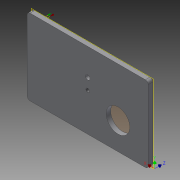
# Autodesk Inventor part: capac
Saved by Autodesk Inventor 2015 SP1 (Build 190203100, 203)
## iProperties
Created: 2015-04-26
Part Number: capac
Material: Generic
Document SubType Name: Modeling
Designer: ubik
Density: 1 g/cm^3
Appearance: Default
Author: ubik
Autodesk Inventor part; units mm, degrees
ref_plane "YZ Plane" through (0, 0, 0) normal (1, 0, 0) x (0, 1, 0)
ref_plane "XZ Plane" through (0, 0, 0) normal (0, 1, 0) x (-1, 0, 0)
ref_plane "XY Plane" through (0, 0, 0) normal (0, 0, 1) x (1, 0, 0)
ref_plane "Work Plane1" through (0, -1.5067, 123.4533) normal (0, 0, 1) x (1, 0, 0)
sketch "Sketch1" plane through (0, -1.5067, 123.4533) normal (0, 0, 1) x (1, 0, 0)
  arc A0 (-98.75, -51) -> (-86.75, -63) centre (-86.75, -51) ccw projected
  line L0 (86.75, -63) -> (-86.75, -63) projected
  arc A1 (86.75, -63) -> (98.75, -51) centre (86.75, -51) ccw projected
  line L1 (98.75, 51) -> (98.75, -51) projected
  arc A2 (98.75, 51) -> (86.75, 63) centre (86.75, 51) ccw projected
  line L2 (-86.75, 63) -> (86.75, 63) projected
  arc A3 (-86.75, 63) -> (-98.75, 51) centre (-86.75, 51) ccw projected
  line L3 (-98.75, -51) -> (-98.75, 51) projected
  line L4 (93.75, 46) -> (93.75, -46) projected
  arc A4 (81.75, -58) -> (93.75, -46) centre (81.75, -46) ccw projected
  line L5 (81.75, -58) -> (-81.75, -58) projected
  arc A5 (-93.75, -46) -> (-81.75, -58) centre (-81.75, -46) ccw projected
  line L6 (-93.75, -46) -> (-93.75, 46) projected
  arc A6 (-81.75, 58) -> (-93.75, 46) centre (-81.75, 46) ccw projected
  line L7 (-81.75, 58) -> (81.75, 58) projected
  arc A7 (93.75, 46) -> (81.75, 58) centre (81.75, 46) ccw projected
  point P0 (0, 1.5067)
sketch "Sketch2" plane through (0, -1.5067, 123.4533) normal (0, 0, 1) x (1, 0, 0)
  line L0 (-107.5, 69.0067) -> (107.5, 69.0067)
  line L1 (107.5, 69.0067) -> (107.5, -65.9933)
  line L2 (107.5, -65.9933) -> (-107.5, -65.9933)
  line L3 (-107.5, -65.9933) -> (-107.5, 69.0067)
  point P0 (0, 1.5067)
  dimension "height" = 135
  dimension "width" = 215
  dimension "d2" = 107.5
  dimension "d3" = 67.5
  constraints: 8 end point, 2 parallel, 1 horizontal, 1 perpendicular
  measures "height" distance of L2.end L0.start
  measures "width" distance of L0.start L0.end
  measures "d2" distance from line of point (0, 1.507) L3
  measures "d3" distance from line of point (0, 1.507) L2
extrude "Extrusion1" add sketch "Sketch2" along normal blind 8
fillet "Fillet1" radius 5 4 edges at (-107.5, 67.5, 127.4533) (107.5, 67.5, 127.4533) (107.5, -67.5, 127.4533) (-107.5, -67.5, 127.4533)
extrude "Extrusion2" cut sketch "Sketch1" along normal blind 3 contours L3 A3 L2 A2 L1 A1 L0 A0 | L4 A4 L5 A5 L6 A6 L7 A7
sketch "Sketch3" plane through (0, -1.5067, 126.4533) normal (0, 0, -1) x (-1, 0, 0)
  line L0 (93.75, 46) -> (93.75, -46)
  arc A0 (81.75, -58) -> (93.75, -46) centre (81.75, -46) ccw
  line L1 (81.75, -58) -> (-81.75, -58)
  arc A1 (-93.75, -46) -> (-81.75, -58) centre (-81.75, -46) ccw
  line L2 (-93.75, -46) -> (-93.75, 46)
  arc A2 (-81.75, 58) -> (-93.75, 46) centre (-81.75, 46) ccw
  line L3 (-81.75, 58) -> (81.75, 58)
  arc A3 (93.75, 46) -> (81.75, 58) centre (81.75, 46) ccw
  point P0 (0, 1.5067)
  point P1 (86.75, -51)
extrude "Extrusion3" add sketch "Sketch3" along normal blind 3
hole "Hole1" at (0, 0, 131.4533) direction (0, 0, -1) diameter 6.647 end through all thread size "M8x1.25" class "6H" standard "ANSI Metric M Profile"
sketch "Sketch4" plane through (0, -1.5067, 123.4533) normal (0, 0, -1) x (-1, 0, 0)
  circle A0 centre (-53.75, -18) radius 37
  line L0 (-15, 6.5067) -> (15, 6.5067)
  line L1 (15, 6.5067) -> (15, 36.5067)
  line L2 (15, 36.5067) -> (-15, 36.5067)
  line L3 (-15, 36.5067) -> (-15, 6.5067)
  line L4 (-93.75, 46) -> (-93.75, -46) projected
  line L5 (-81.75, -58) -> (81.75, -58) projected
  circle A1 centre (-53.75, -18) radius 21
  point P0 (0, 1.5067)
  dimension "d20" = 74
  dimension "d21" = 30
  dimension "d22" = 30
  dimension "d23" = 15
  dimension "d24" = 40
  dimension "d25" = 40
  dimension "d26" = 5
  dimension "d27" = 42
  constraints: 8 end point, 2 centre point, 2 parallel, 1 coincident, 1 horizontal, 1 perpendicular
  measures "d20" diameter of A0
  measures "d21" distance of L2.end L1.end
  measures "d22" distance of L1.end L0.end
  measures "d23" distance from line of point (0, 1.507) L3
  measures "d24" distance from line of A0.centre L4
  measures "d25" distance from line of A0.centre L5
  measures "d26" distance from line of point (0, 1.507) L0
  measures "d27" diameter of A1
extrude "Extrusion4" cut sketch "Sketch4" against normal through all contours A1
hole "Hole2" at (0, 20, 123.4533) direction (0, 0, 1) diameter 8 end through all
equation "\"d2\" = 0.5 * width"
equation "\"d3\" = 0.5 * height"
equation "\"d9\" = 0.5 * height"
equation "\"d10\" = 0.5 * width"
equation "\"d30\" = 0.5 * width"
body "Solid1"
